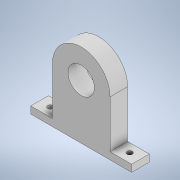
# Autodesk Inventor part: sopoetellantas
Saved by Autodesk Inventor 2021 (Build 250183000, 183)
## iProperties
Created: 2021-02-06
Part Number: sopoetellantas
Material: Genérico
Document SubType Name: Modeling
Designer: jaime
Density: 1 g/cm^3
Appearance: Valor por defecto
Author: jaime
Autodesk Inventor part; units mm, degrees
ref_plane "YZ Plane" through (0, 0, 0) normal (1, 0, 0) x (0, 1, 0)
ref_plane "XZ Plane" through (0, 0, 0) normal (0, 1, 0) x (-1, 0, 0)
ref_plane "XY Plane" through (0, 0, 0) normal (0, 0, 1) x (1, 0, 0)
sketch "Boceto1" plane through (0, 0, 0) normal (0, 0, 1) x (1, 0, 0)
  arc A0 (0, 16.3821) -> (-16.3821, 0) centre (0, 0) ccw
  line L0 (-16.3821, 0) -> (-16.3821, -26.9516)
  line L1 (-16.3821, -26.9516) -> (-28.6667, -26.9516)
  line L2 (-28.6667, -26.9516) -> (-28.6667, -30.9943)
  line L3 (-28.6667, -30.9943) -> (0, -30.9943)
  line L4 (0, -30.9943) -> (0, 16.3821) construction
  arc A1 (0, 7.5) -> (0, -7.5) centre (0, 0) ccw
  arc A2 (16.3821, 0) -> (0, 16.3821) centre (0, 0) ccw
  line L5 (16.3821, 0) -> (16.3821, -26.9516)
  line L6 (16.3821, -26.9516) -> (28.6667, -26.9516)
  line L7 (28.6667, -26.9516) -> (28.6667, -30.9943)
  line L8 (28.6667, -30.9943) -> (0, -30.9943)
  arc A3 (0, -7.5) -> (0, 7.5) centre (0, 0) ccw
  dimension "d2" = 7.5
  constraints: 18 end point, 8 point on circle, 4 centre point, 4 symmetric about line, 3 coincident, 3 vertical, 2 point on line, 1 horizontal, 1 perpendicular, 1 tangent, 2 other
  measures "d2" radius of A1
extrude "Extrusión1" add sketch "Boceto1" along normal blind 10
sketch "Boceto2" plane through (-28.6667, -26.9516, 0) normal (0, 1, 0) x (1, 0, 0)
  line L0 (12.2846, 0) -> (45.0488, 0) projected
  line L1 (0, -10) -> (57.3334, -10) projected
  line L2 (12.2846, 0) -> (0, -10)
  line L3 (12.2846, -10) -> (45.0488, -10) projected
  line L4 (0, 0) -> (57.3334, 0) projected
  line L5 (12.2846, -10) -> (0, 0)
  line L6 (0, 0) -> (57.3334, -10)
  line L7 (0, -10) -> (57.3334, 0)
  line L8 (28.6667, -5) -> (28.6667, 11.6359)
  circle A0 centre (6.1423, -5) radius 1.5
  circle A1 centre (51.1911, -5) radius 1.5
  point P0 (28.6667, 0)
  dimension "d3" = 3
  constraints: 10 end point, 2 centre point, 2 midpoint, 1 symmetric about line, 1 vertical, 1 other
  measures "d3" diameter of A0
extrude "Extrusión2" cut sketch "Boceto2" against normal blind 5 contours A0 L5 L2 | L2 L5 A0 | L5 L2 A0 | L5 A0 L2 | A1
